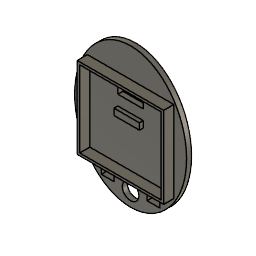
Panel1 (Autodesk Fusion 360 design; units mm, degrees)
part number: 2026-05-23-22-37-07-579
Autodesk Fusion 360 part; units mm, degrees
sketch "Sketch1" plane through (0, 0, 0) normal (0, 1, 0) x (1, 0, 0)
  ellipse E0 centre (0, 0) end of major axis (0, 27.5) minor radius 22
  line L0 (0, -27.5) -> (0, 27.5) construction
  line L1 (22, 0) -> (-22, 0) construction
  dimension "d34" = 55
  dimension "d35" = 44
  constraint coincident E0 L0.start
  constraint coincident E0 L0.end
  constraint coincident E0 L1.start
  constraint coincident E0 L1.end
  constraint coincident E0.centre origin
  constraint vertical L0
  measures "d34" distance of E0
extrude "Extrude1" add sketch "Sketch1" along normal blind 2 makes body 1
sketch "Sketch2" plane through (0, 0, 0) normal (0, -1, 0) x (1, 0, 0)
  line L0 (-17, 16) -> (17, 16)
  line L1 (17, 16) -> (17, -16)
  line L2 (17, -16) -> (-17, -16)
  line L3 (-17, -16) -> (-17, 16)
  line L4 (-16, 15) -> (16, 15)
  line L5 (16, 15) -> (16, -15)
  line L6 (16, -15) -> (-16, -15)
  line L7 (-16, -15) -> (-16, 15)
  ellipse E0 centre (0, 0) end of major axis (0, -27.5) minor radius 22
  point P0 (-9.0615, 23.3)
  point P1 (0, 27.5)
  point P2 (0, -27.5)
  dimension "d5" = 1
  dimension "d6" = 1
  dimension "d7" = 1
  dimension "d8" = 1
  dimension "d45" = 34
  dimension "d46" = 32
  dimension "d47" = 12.5
  dimension "d48" = 12.5
  constraint horizontal L0
  constraint vertical L1
  constraint horizontal L2
  constraint vertical L3
  constraint horizontal L4
  constraint vertical L5
  constraint horizontal L6
  constraint vertical L7
  constraint coincident E0 P1
  constraint coincident E0 P2
  measures "d5" distance of L0 L4
  measures "d6" distance of L1 L5
  measures "d7" distance of L2 L6
  measures "d8" distance of L3 L7
  measures "d45" distance of L0.start L0.end
  measures "d46" distance of L0.end L1.end
  measures "d47" distance of L4 P1
  measures "d48" distance of L6 P2
extrude "Extrude2" add sketch "Sketch2" along normal blind 4 separate body contours L0 L1 L2 L3 makes body 2
sketch "Sketch3" plane through (0, 0, 0) normal (0, -1, 0) x (1, 0, 0)
  line L0 (-5, 11) -> (5, 11)
  line L1 (5, 11) -> (5, 8.5)
  line L2 (5, 8.5) -> (-5, 8.5)
  line L3 (-5, 8.5) -> (-5, 11)
  line L4 (-16, 15) -> (16, 15)
  line L5 (-5, 4.5) -> (5, 4.5)
  line L6 (5, 4.5) -> (5, 2)
  line L7 (5, 2) -> (-5, 2)
  line L8 (-5, 2) -> (-5, 4.5)
  ellipse E0 centre (0, 0) end of major axis (0, -27.5) minor radius 22
  dimension "d11" = 2.5
  dimension "d12" = 10
  dimension "d13" = 4
  dimension "d14" = 2.5
  dimension "d15" = 10
  dimension "d16" = 4
  constraint horizontal L0
  constraint vertical L1
  constraint horizontal L2
  constraint vertical L3
  constraint horizontal L5
  constraint vertical L6
  constraint horizontal L7
  constraint vertical L8
  measures "d11" distance of L0.start L2.end
  measures "d12" distance of L0.start L0.end
  measures "d13" distance of L0 L4
  measures "d14" distance of L5.start L7.end
  measures "d15" distance of L6.end L7.end
  measures "d16" distance of L2 L5
extrude "Extrude3" cut sketch "Sketch3" against normal blind 12 contours L0 L1 L2 L3 bodies 1
extrude "Extrude4" add sketch "Sketch3" along normal blind 1.5 contours L5 L6 L7 L8 bodies 1
sketch "Sketch5" plane through (0, 0, 0) normal (0, -1, 0) x (1, 0, 0)
  line L0 (-5, 2) -> (-5, 4.5)
  line L1 (-5, 4.5) -> (5, 4.5)
  line L2 (5, 4.5) -> (5, 2)
  line L3 (5, 2) -> (-5, 2)
  line L4 (5, 11) -> (5, 8.5)
  line L5 (5, 8.5) -> (-5, 8.5)
  line L6 (-5, 8.5) -> (-5, 11)
  line L7 (-5, 11) -> (5, 11)
  ellipse E0 centre (0, 0) end of major axis (0, -27.5) minor radius 22
  line L8 (-11.5, -17) -> (-6.5, -17)
  line L9 (-6.5, -17) -> (-6.5, -22)
  line L10 (-6.5, -22) -> (-11.5, -22)
  line L11 (-11.5, -22) -> (-11.5, -17)
  line L12 (-17, -16) -> (17, -16)
  line L13 (6.5, -17) -> (11.5, -17)
  line L14 (11.5, -17) -> (11.5, -22)
  line L15 (11.5, -22) -> (6.5, -22)
  line L16 (6.5, -22) -> (6.5, -17)
  circle A0 centre (0, -22) radius 3.25
  line L17 (-17, -16) -> (-17, -24.6969) construction
  line L18 (17, -16) -> (17, -29.3033) construction
  dimension "d36" = 5
  dimension "d37" = 5
  dimension "d38" = 1
  dimension "d39" = 5
  dimension "d40" = 5
  dimension "d41" = 1
  dimension "d42" = 13
  dimension "d43" = 6.5
  dimension "d44" = 6
  dimension "d49" = 5.5
  dimension "d50" = 5.5
  constraint horizontal L8
  constraint vertical L9
  constraint horizontal L10
  constraint vertical L11
  constraint horizontal L13
  constraint vertical L14
  constraint horizontal L15
  constraint vertical L16
  constraint coincident L12.start L17.start
  constraint perpendicular L12 L17
  constraint coincident L12.end L18.start
  constraint perpendicular L12 L18
  measures "d36" distance of L8.start L8.end
  measures "d37" distance of L8.start L10.end
  measures "d38" distance of L8 L12
  measures "d39" distance of L13.start L13.end
  measures "d40" distance of L13.start L15.end
  measures "d41" distance of L12 L13
  measures "d42" distance of L9 L16
  measures "d43" diameter of A0
  measures "d44" distance of L12 A0.centre
  measures "d49" distance of L14 L18
  measures "d50" distance of L11 L17
extrude "Extrude7" cut sketch "Sketch5" against normal blind 9 contours L8 L9 L10 L11 | L13 L14 L15 L16 | A0 bodies 1
